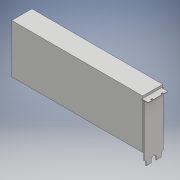
# Autodesk Inventor part: Vega56dummy
Saved by Autodesk Inventor 2017 (Build 210142000, 142)
## iProperties
Created: 2019-06-28
Part Number: Vega56dummy
Material: Generic
Document SubType Name: Modeling
Designer: DDeGo
Density: 1 g/cm^3
Appearance: Default
Author: DDeGo
Autodesk Inventor part; units mm, degrees
ref_plane "YZ Plane" through (0, 0, 0) normal (1, 0, 0) x (0, 1, 0)
ref_plane "XZ Plane" through (0, 0, 0) normal (0, 1, 0) x (-1, 0, 0)
ref_plane "XY Plane" through (0, 0, 0) normal (0, 0, 1) x (1, 0, 0)
sketch "Sketch1" plane through (0, 0, 0) normal (1, 0, 0) x (0, 1, 0)
  line L0 (0, 0) -> (40.8, 0)
  line L1 (40.8, 0) -> (40.8, 99)
  line L2 (40.8, 99) -> (0, 99)
  line L3 (0, 99) -> (0, 0)
  dimension "d0" = 40.8
  dimension "d1" = 99
  constraints: 8 end point, 2 parallel, 1 horizontal, 1 perpendicular
  measures "d0" distance of L1.end L2.end
  measures "d1" distance between parallel lines of L0 L2
extrude "Extrusion1" add sketch "Sketch1" along normal blind 265
sketch "Sketch2" plane through (265, 0, 0) normal (1, 0, 0) x (0, 0, -1)
  line L0 (0, 40.8) -> (-99, 40.8) projected
  line L1 (-94.5, 40.8) -> (-94.5, -1.5)
  line L2 (-94.5, -1.5) -> (-93.5, -1.5)
  line L3 (-93.5, -1.5) -> (-93.5, 1.8)
  line L4 (-93.5, 1.8) -> (14.5, 1.8)
  line L5 (14.5, 1.8) -> (18.5, 5.8)
  line L6 (18.5, 5.8) -> (26, 5.8)
  line L7 (26, 5.8) -> (26, 16.3)
  line L8 (26, 16.3) -> (18.5, 16.3)
  line L9 (18.5, 16.3) -> (14.5, 21.3)
  line L10 (14.5, 21.3) -> (18.5, 26.3)
  line L11 (18.5, 26.3) -> (26, 26.3)
  line L12 (26, 26.3) -> (26, 36.8)
  line L13 (26, 36.8) -> (18.5, 36.8)
  line L14 (18.5, 36.8) -> (14.5, 40.8)
  line L15 (14.5, 40.8) -> (0, 40.8)
  line L16 (0, 0) -> (0, 40.8) projected
  line L17 (0, 40.8) -> (-94.5, 40.8)
  line L18 (-99, 40.8) -> (-99, 0) projected
  line L19 (-99, 0) -> (0, 0) projected
  line L20 (14.5, 21.3) -> (14.5, 40.8) construction
  dimension "d4" = 4.5
  dimension "d5" = 1
  dimension "d6" = 1.5
  dimension "d7" = 135
  dimension "d8" = 135
  dimension "d9" = 10.5
  dimension "d10" = 4
  dimension "d11" = 7.5
  dimension "d13" = 10
  dimension "d14" = 108
  constraints: 34 end point, 8 perpendicular, 6 equal length, 2 horizontal, 2 vertical, 1 collinear, 1 parallel, 1 point on line
  measures "d4" distance between parallel lines of L18 L1
  measures "d5" distance between parallel lines of L1 L3
  measures "d6" distance from line of L2.end L19
  measures "d7" angle of L15 L14
  measures "d8" angle of L4 L5
  measures "d9" distance of L11.end L12.end
  measures "d10" distance between parallel lines of L4 L6
  measures "d11" distance of L12.end L13.end
  measures "d13" distance between parallel lines of L8 L11
  measures "d14" distance between parallel lines of L3 L20
extrude "Extrusion2" add sketch "Sketch2" along normal blind 1 contours L16 L4 L3 L19 L1 L0 | L15 L14 L13 L12 L11 L10 L9 L8 L7 L6 L5 L4 L16 | L19 L3 L2 L1
sketch "Sketch3" plane through (265, -1.5, 94.5) normal (0, 0, 1) x (1, 0, 0)
  line L0 (1, 42.3) -> (1, 0) projected
  line L1 (1, 0) -> (12.5, 0)
  line L2 (12.5, 0) -> (12.5, 8.05)
  line L3 (12.5, 8.05) -> (9.5, 8.05)
  line L4 (9.5, 8.05) -> (9.5, 11.05)
  line L5 (9.5, 11.05) -> (12.5, 11.05)
  line L6 (12.5, 11.05) -> (12.5, 28.55)
  line L7 (12.5, 28.55) -> (9.5, 28.55)
  line L8 (9.5, 28.55) -> (9.5, 31.55)
  line L9 (9.5, 31.55) -> (12.5, 31.55)
  line L10 (12.5, 31.55) -> (12.5, 39.7)
  line L11 (12.5, 39.7) -> (1, 39.7)
  line L12 (1, 39.7) -> (1, 0)
  line L13 (0, 42.3) -> (0, 1.5) projected
  line L14 (0, 42.3) -> (1, 42.3) projected
  point P0 (-265, 1.5)
  point P1 (9.5, 30.05)
  point P2 (9.5, 9.55)
  dimension "d17" = 11.5
  dimension "d18" = 12.25
  dimension "d19" = 20.5
  dimension "d20" = 3
  dimension "d21" = 3
  dimension "d22" = 3
  dimension "d23" = 2.6
  constraints: 24 end point, 7 perpendicular, 7 point on line, 2 midpoint, 1 horizontal, 1 parallel
  measures "d17" distance of L0.end L1.end
  measures "d18" distance from line of point (9.5, 30.05) L14
  measures "d19" distance of point (9.5, 9.55) point (9.5, 30.05)
  measures "d20" distance between parallel lines of L5 L3
  measures "d21" distance between parallel lines of L9 L7
  measures "d22" distance between parallel lines of L8 L6
  measures "d23" distance between parallel lines of L14 L11
extrude "Extrusion3" add sketch "Sketch3" against normal blind 1
body "Solid1"
